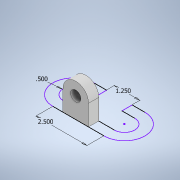
# Autodesk Inventor part: CouplingBase
Saved by Autodesk Inventor 2022.2 (Build 262287030, 287C)
## iProperties
Created: 2023-02-22
Part Number: CouplingBase
Material: Generic
Document SubType Name: Modeling
Designer: jak27277
Density: 1 g/cm^3
Appearance: Default
Author: jak27277
Autodesk Inventor part; units mm, degrees
ref_plane "YZ Plane" through (0, 0, 0) normal (1, 0, 0) x (0, 1, 0)
ref_plane "XZ Plane" through (0, 0, 0) normal (0, 1, 0) x (-1, 0, 0)
ref_plane "XY Plane" through (0, 0, 0) normal (0, 0, 1) x (1, 0, 0)
sketch "Sketch2" plane through (0, 0, 0) normal (0, 0, 1) x (1, 0, 0)
  circle A0 centre (0, 0) radius 6.35
  arc A1 (15.875, 0) -> (-15.875, 0) centre (0, 0) ccw
  line L0 (-15.875, 0) -> (-15.875, -25.4)
  line L1 (-15.875, -25.4) -> (15.875, -25.4)
  line L2 (15.875, -25.4) -> (15.875, 0)
  dimension "d0" = 15.875
  dimension "d1" = 25.4
  dimension "d2" = 12.7
  constraints: 6 end point, 2 centre point, 2 coincident, 2 point on circle, 2 tangent, 2 vertical, 1 perpendicular
  measures "d0" radius of A1
  measures "d1" distance of L0.start L0.end
  measures "d2" diameter of A0
extrude "Extrusion1" add sketch "Sketch2" along normal blind 12.7
sketch "Sketch3" plane through (-15.875, -25.4, 0) normal (0, -1, 0) x (1, 0, 0)
  line L0 (0, 0) -> (31.75, 0) projected
  line L1 (50.8718, 12.7) -> (-12.6282, 12.7)
  arc A0 (50.8718, -38.1) -> (50.8718, 12.7) centre (50.8718, -12.7) ccw
  arc A1 (-12.6282, 12.7) -> (-11.6213, -38.08) centre (-12.6282, -12.7) ccw
  arc A2 (50.8718, -25.4) -> (50.8718, 0) centre (50.8718, -12.7) ccw
  arc A3 (-12.6282, 0) -> (-12.6282, -25.4) centre (-12.6282, -12.7) ccw
  line L2 (50.8718, 0) -> (-12.6282, 0)
  line L3 (0, 12.7) -> (31.75, 12.7) projected
  line L4 (50.8718, -25.4) -> (34.9968, -25.4)
  line L5 (34.9968, -25.4) -> (34.9968, -38.1)
  line L6 (34.9968, -38.1) -> (50.8718, -38.1)
  line L7 (-12.6282, -25.4) -> (3.2468, -25.4)
  line L8 (3.2468, -25.4) -> (3.2468, -38.1)
  line L9 (3.2468, -38.1) -> (-12.6282, -38.1)
  line L10 (9.525, 12.7) -> (22.225, 12.7) projected
  line L11 (9.525, 0) -> (22.225, 0) projected
  line L12 (9.525, 0) -> (22.225, 0) projected
  point P0 (15.875, 0)
  dimension "d6" = 63.5
  dimension "d7" = 12.7
  dimension "d9" = 31.75
  constraints: 16 end point, 9 point on circle, 6 tangent, 4 centre point, 3 collinear, 3 horizontal, 3 perpendicular, 3 point on line, 2 coincident, 1 equal radius
  measures "d6" distance of L1.start L1.end
  measures "d7" radius of A3
  measures "d9" distance between parallel lines of L8 L5
body "Solid1"
